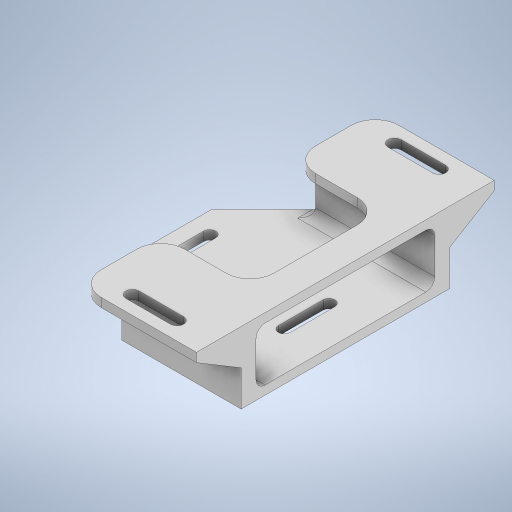
# Autodesk Inventor part: soporte infe
Saved by Autodesk Inventor 2024 (Build 280153000, 153)
## iProperties
Created: 2024-04-18
Part Number: soporte infe
Material: Generic
Document SubType Name: Modeling
Designer: compu
Density: 1 g/cm^3
Appearance: Default
Author: compu
Autodesk Inventor part; units mm, degrees
ref_plane "YZ Plane" through (0, 0, 0) normal (1, 0, 0) x (0, 1, 0)
ref_plane "XZ Plane" through (0, 0, 0) normal (0, 1, 0) x (-1, 0, 0)
ref_plane "XY Plane" through (0, 0, 0) normal (0, 0, 1) x (1, 0, 0)
sketch "Sketch1" plane through (0, 0, 0) normal (0, 1, 0) x (-1, 0, 0)
  line L0 (8, 0) -> (-48, 0) projected
  line L1 (0, -70) -> (0, 70) projected
  line L2 (-40, 50) -> (0, 50)
  line L3 (0, 50) -> (0, -50)
  line L4 (0, -50) -> (-40, -50)
  line L5 (-40, -50) -> (-40, 50)
  point P0 (0, 0)
  point P1 (0, 50)
  dimension "d0" = 40
  dimension "d1" = 100
  constraints: 8 end point, 2 parallel, 1 collinear, 1 horizontal, 1 perpendicular, 1 other
  measures "d0" distance of L3.end L4.end
  measures "d1" distance of L2.end L3.end
extrude "Extrusion1" add sketch "Sketch1" against normal blind 3
sketch "Sketch2" plane through (0, -3, 0) normal (0, -1, 0) x (1, 0, 0)
  line L0 (0, -50) -> (40, -50) projected
  line L1 (40, -50) -> (40, 50) projected
  line L2 (40, 50) -> (0, 50) projected
  line L3 (0, 50) -> (0, -50) projected
  line L4 (40, 35) -> (0, 35)
  line L5 (40, -50) -> (40, 50) projected
  line L6 (40, -35) -> (0, -35)
  line L7 (40, 30) -> (0, 30)
  line L8 (40, -30) -> (0, -30)
  point P0 (0, 0)
  dimension "d4" = 15
  dimension "d5" = 15
  dimension "d6" = 5
  dimension "d7" = 5
  constraints: 8 end point, 8 point on line, 4 perpendicular
  measures "d4" distance between parallel lines of L2 L4
  measures "d5" distance between parallel lines of L0 L6
  measures "d6" distance between parallel lines of L4 L7
  measures "d7" distance between parallel lines of L6 L8
extrude "Extrusion2" add sketch "Sketch2" along normal blind 21 contours L3 L8 L1 L6 | L3 L4 L1 L7
sketch "Sketch3" plane through (0, 0, 0) normal (0, 1, 0) x (1, 0, 0)
  line L0 (40, 50) -> (0, 50) projected
  line L1 (0, 50) -> (0, -50) projected
  line L2 (0, -50) -> (40, -50) projected
  line L3 (40, -50) -> (40, 50) projected
  line L4 (0, -44) -> (40, -44) construction
  arc A0 (12.5, -41.8) -> (12.5, -46.2) centre (12.5, -44) ccw
  arc A1 (27.5, -46.2) -> (27.5, -41.8) centre (27.5, -44) ccw
  line L5 (12.5, -41.8) -> (27.5, -41.8)
  line L6 (12.5, -46.2) -> (27.5, -46.2)
  line L7 (-8, 0) -> (48, 0) projected
  arc A2 (12.5, 46.2) -> (12.5, 41.8) centre (12.5, 44) ccw
  arc A3 (27.5, 41.8) -> (27.5, 46.2) centre (27.5, 44) ccw
  line L8 (12.5, 41.8) -> (27.5, 41.8)
  line L9 (12.5, 46.2) -> (27.5, 46.2)
  point P0 (0, 0)
  dimension "d10" = 6
  dimension "d11" = 4.4
  dimension "d12" = 4.4
  dimension "d13" = 15
  dimension "d14" = 12.5
  constraints: 10 end point, 8 point on circle, 6 symmetric about line, 4 centre point, 4 point on line, 2 horizontal, 2 tangent, 1 perpendicular, 2 other
  measures "d10" distance between parallel lines of L2 L4
  measures "d11" diameter of A0
  measures "d12" diameter of A1
  measures "d13" distance of A1.centre A0.centre
  measures "d14" distance from line of L3 A1.centre
extrude "Extrusion3" cut sketch "Sketch3" against normal blind 18 contours L5 A1 L6 A0 | L9 A3 L8 A2
sketch "Sketch4" plane through (0, -24, 0) normal (0, -1, 0) x (1, 0, 0)
  line L0 (40, 35) -> (-20, 35)
  line L1 (-20, 35) -> (-20, -35)
  line L2 (-20, -35) -> (40, -35)
  line L3 (40, -35) -> (40, 35)
  line L4 (40, 30) -> (40, 35) projected
  line L5 (40, 35) -> (0, 35) projected
  line L6 (0, 35) -> (0, 30) projected
  line L7 (0, 30) -> (40, 30) projected
  line L8 (0, -30) -> (0, -35) projected
  line L9 (0, -35) -> (40, -35) projected
  line L10 (40, -35) -> (40, -30) projected
  line L11 (40, -30) -> (0, -30) projected
  line L12 (40, 35) -> (0, 35) projected
  line L13 (0, -35) -> (40, -35) projected
  line L14 (40, -30) -> (40, 30) projected
  line L15 (40, -35) -> (40, -30) projected
  point P0 (0, 0)
  dimension "d18" = 20
  constraints: 8 end point, 3 collinear, 2 parallel, 1 horizontal, 1 perpendicular
  measures "d18" distance between parallel lines of L8 L1
extrude "Extrusion4" add sketch "Sketch4" against normal blind 3
sketch "Sketch5" plane through (0, 0, 0) normal (0, 1, 0) x (1, 0, 0)
  arc A0 (27.5, 41.8) -> (27.5, 46.2) centre (27.5, 44) ccw projected
  line L0 (27.5, 41.8) -> (12.5, 41.8) projected
  arc A1 (12.5, 46.2) -> (12.5, 41.8) centre (12.5, 44) ccw projected
  line L1 (12.5, 46.2) -> (27.5, 46.2) projected
  arc A2 (27.5, -46.2) -> (27.5, -41.8) centre (27.5, -44) ccw projected
  line L2 (27.5, -46.2) -> (12.5, -46.2) projected
  arc A3 (12.5, -41.8) -> (12.5, -46.2) centre (12.5, -44) ccw projected
  line L3 (12.5, -41.8) -> (27.5, -41.8) projected
  line L4 (40, 50) -> (0, 50) projected
  line L5 (0, 50) -> (0, -50) projected
  line L6 (0, -50) -> (40, -50) projected
  line L7 (40, -50) -> (40, 50) projected
  line L8 (-9.315, 0) -> (55.8902, 0) projected
  line L9 (40, -30) -> (0, -30) projected
  line L10 (0, 30) -> (40, 30) projected
  line L11 (40, -30) -> (40, 0) construction
  line L12 (40, 30) -> (40, 0) construction
  line L13 (0, -22) -> (30, -22)
  line L14 (30, -22) -> (30, 22)
  line L15 (30, 22) -> (0, 22)
  line L16 (0, 22) -> (0, -22)
  point P0 (0, 0)
  point P1 (0, 22)
  dimension "d30" = 44
  dimension "d31" = 10
  constraints: 12 end point, 2 parallel, 2 perpendicular, 2 point on line, 1 horizontal, 1 midpoint, 1 other
  measures "d30" distance of L13.end L14.end
  measures "d31" distance between parallel lines of L12 L14
extrude "Extrusion5" cut sketch "Sketch5" against normal up to surface (21 mm away) contours L15 L14 L8 L5 | L14 L13 L5 L8
sketch "Sketch6" plane through (40, -3, 50) normal (1, 0, 0) x (0, 0, -1)
  line L0 (0, 3) -> (100, 3) projected
  line L1 (0, 3) -> (0, 0) projected
  line L2 (15, 0) -> (0, 0) projected
  line L3 (15, 0) -> (15, -21) projected
  line L4 (85, -21) -> (15, -21) projected
  line L5 (85, 0) -> (85, -21) projected
  line L6 (100, 0) -> (85, 0) projected
  line L7 (100, 3) -> (100, 0) projected
  line L8 (80, 0) -> (20, 0) projected
  line L9 (80, 0) -> (80, -18) projected
  line L10 (20, -18) -> (80, -18) projected
  line L11 (20, 0) -> (20, -18) projected
  line L12 (85, 0) -> (85, -21)
  line L13 (100, 0) -> (85, 0)
  line L14 (0, 0) -> (15, 0)
  line L15 (3.8, 3) -> (3.8, 0) projected
  line L16 (15, -21) -> (15, 0)
  line L17 (0, 0) -> (15, -9)
  line L18 (15, 0) -> (15, -21) projected
  line L19 (100, 0) -> (85, -9)
  line L20 (85, 0) -> (85, -21) projected
  point P0 (50, 3)
  dimension "d53" = 12
  dimension "d54" = 12
  constraints: 12 end point, 2 collinear, 2 perpendicular, 2 point on line
  measures "d53" distance of L3.end L17.end
  measures "d54" distance of L4.start L19.end
extrude "Extrusion6" add sketch "Sketch6" against normal blind 3 contours L2 L3 L17 | L19 L5 L6
fillet "Fillet1" radius 8 4 edges at (30, -1.5, 22) (30, -1.5, -22) (0, -1.5, -22) (0, -1.5, 22)
chamfer "Chamfer1" distance 20 angle 45 2 edges at (-20, -22.5, -35) (-20, -22.5, 35)
sketch "Sketch9" plane through (0, -21, 0) normal (0, 1, 0) x (1, 0, 0)
  line L0 (-32, 0) -> (52, 0) projected
  line L1 (0, 70) -> (0, -70) projected
  line L2 (-20, 15) -> (-20, -15) projected
  arc A0 (-15, -7.5) -> (-11, -7.5) centre (-13, -7.5) ccw
  arc A1 (-11, 7.5) -> (-15, 7.5) centre (-13, 7.5) ccw
  line L3 (-13, -15) -> (-13, 15) construction
  line L4 (-15, -7.5) -> (-15, 7.5)
  line L5 (-11, -7.5) -> (-11, 7.5)
  arc A2 (25, -7.5) -> (29, -7.5) centre (27, -7.5) ccw
  arc A3 (29, 7.5) -> (25, 7.5) centre (27, 7.5) ccw
  line L6 (25, -7.5) -> (25, 7.5)
  line L7 (29, -7.5) -> (29, 7.5)
  point P0 (0, 0)
  dimension "d36" = 4
  dimension "d37" = 4
  dimension "d38" = 15
  dimension "d40" = 7
  dimension "d41" = 7.5
  dimension "d42" = 4
  dimension "d43" = 4
  dimension "d44" = 15
  dimension "d45" = 40
  dimension "d46" = 7.5
  constraints: 10 end point, 8 point on circle, 5 vertical, 4 centre point, 4 tangent, 2 point on line
  measures "d36" diameter of A0
  measures "d37" diameter of A1
  measures "d38" distance of A1.centre A0.centre
  measures "d40" distance between parallel lines of L2 L3
  measures "d41" distance from line of L0 A1.centre
  measures "d42" diameter of A2
  measures "d43" diameter of A3
  measures "d44" distance of A3.centre A2.centre
  measures "d45" distance of A3.centre A1.centre
  measures "d46" distance from line of L0 A3.centre
extrude "Extrusion9" cut sketch "Sketch9" against normal blind 10
fillet "Fillet2" radius 8 1 edges at (0, -1.5, -50)
fillet "Fillet3" radius 8 1 edges at (0, -1.5, 50)
fillet "Fillet4" radius 3 8 edges at (20, -21, -30) (0, -21, -32.5) (20, -21, 30) (0, -21, 32.5) (18.5, -3, 35) (20, -3, 30) (18.5, -3, -35) (20, -3, -30)
body "Solid1"
